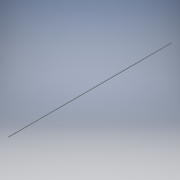
# Autodesk Inventor part: Slotted center beam_xw
Saved by Autodesk Inventor 2016 (Build 200138000, 138)
## iProperties
Created: 2013-10-22
Part Number: Slotted center beam_xw
Document SubType Name: Modeling
Designer: 121767
Density: 1 g/cm^3
Material: Generic
Appearance: Default
Author: 121767
Autodesk Inventor part; units mm, degrees
ref_plane "YZ Plane" through (0, 0, 0) normal (1, 0, 0) x (0, 1, 0)
ref_plane "XZ Plane" through (0, 0, 0) normal (0, 1, 0) x (-1, 0, 0)
ref_plane "XY Plane" through (0, 0, 0) normal (0, 0, 1) x (1, 0, 0)
sketch "Sketch1" plane through (0, 0, 0) normal (0, 0, 1) x (1, 0, 0)
  line L0 (-2.54, -3.0539) -> (-2.54, -1.905)
  line L1 (-2.54, -1.905) -> (2.54, -1.905)
  line L2 (2.54, -1.905) -> (2.54, -3.0539)
  arc A0 (2.54, -3.0539) -> (-2.54, -3.0539) centre (0, 0) ccw
  line L3 (0, -1.905) -> (0, -6.1579) construction
  arc A1 (-2.3876, 2.4839) -> (2.3876, 2.4839) centre (0, 2.4839) ccw
  line L4 (0, 2.4839) -> (2.3876, 2.4839) construction
  line L5 (0, 2.4839) -> (-2.3876, 2.4839) construction
  line L6 (-2.3876, 2.4839) -> (-2.3876, 3.1745)
  line L7 (2.3876, 2.4839) -> (2.3876, 3.1745)
  point P0 (-2.54, -1.905)
  point P1 (2.54, -1.905)
  dimension "d14" = 5.08
  dimension "d22" = 2.3876
  dimension "d23" = 180
  constraints: 16 end point, 6 point on circle, 3 parallel, 2 centre point, 2 point on line, 2 tangent, 1 coincident, 1 midpoint, 1 vertical, 1 other
  measures "d14" distance between parallel lines of L2 L0
  measures "d22" radius of A1
  measures "d23" angle of L5 L4
extrude "Extrusion4" add sketch "Sketch1" along normal blind 2438.4 contours A0 L6 A1 L7 L2 L1 L0
sketch "Sketch2" plane through (0, 0, 0) normal (0, 0, -1) x (-1, 0, 0)
  line L0 (2.54, -3.0539) -> (2.54, -1.905) projected
  line L1 (-2.54, -1.905) -> (-2.54, -3.0539) projected
  line L2 (2.54, -3.0539) -> (2.54, -1.905) projected
  line L3 (2.54, -1.905) -> (2.54, 0.3497)
  line L4 (2.54, 0.3497) -> (-2.54, 0.3497)
  line L5 (-2.54, -1.905) -> (-2.54, -3.0539) projected
  line L6 (-2.54, 0.3497) -> (-2.54, -1.905)
  point P0 (0, 0)
  dimension "d24" = 3.4036
  constraints: 6 end point, 2 collinear, 2 perpendicular, 1 vertical
  measures "d24" distance of L3.end L0.start
extrude "Extrusion5" cut sketch "Sketch2" against normal blind 15 fills toward (2.49, -0.7776) open curves L3 L4 L6
body "Solid3"
